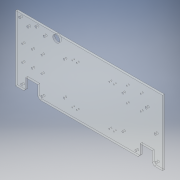
# Autodesk Inventor part: LexanPlatebkp
Saved by Autodesk Inventor 2018 (Build 220112000, 112)
## iProperties
Created: 2017-09-07
Part Number: LexanPlatebkp
Material: Polycarbonate, Clear
Document SubType Name: Modeling
Designer: Srinity
Density: 1.2 g/cm^3
Appearance: Polycarbonate - Clear
Author: Srinity
Autodesk Inventor part; units mm, degrees
ref_plane "YZ Plane" through (0, 0, 0) normal (1, 0, 0) x (0, 1, 0)
ref_plane "XZ Plane" through (0, 0, 0) normal (0, 1, 0) x (-1, 0, 0)
ref_plane "XY Plane" through (0, 0, 0) normal (0, 0, 1) x (1, 0, 0)
sketch "Sketch1" plane through (0, 0, 0) normal (0, 0, 1) x (1, 0, 0)
  line L0 (-228.6, 101.6) -> (228.6, 101.6)
  line L1 (228.6, 101.6) -> (228.6, -101.6)
  line L2 (228.6, -101.6) -> (-228.6, -101.6)
  line L3 (-228.6, -101.6) -> (-228.6, 101.6)
  point P0 (0, 0)
  dimension "d0" = 457.2
  dimension "d1" = 203.2
  dimension "d2" = 228.6
  dimension "d3" = 101.6
  constraints: 8 end point, 2 parallel, 1 horizontal, 1 perpendicular
  measures "d0" distance of L0.start L0.end
  measures "d1" distance of L2.end L0.start
  measures "d2" distance from line of point (0, 0) L3
  measures "d3" distance from line of point (0, 0) L0
extrude "Extrusion1" add sketch "Sketch1" along normal blind 6.35
sketch "Sketch2" plane through (0, 0, 6.35) normal (0, 0, 1) x (1, 0, 0)
  line L0 (-228.6, -101.6) -> (228.6, -101.6) projected
  line L1 (-196.85, -101.6) -> (-158.75, -101.6)
  line L2 (-158.75, -101.6) -> (-158.75, -63.5)
  line L3 (-158.75, -63.5) -> (-196.85, -63.5)
  line L4 (-196.85, -63.5) -> (-196.85, -101.6)
  line L5 (158.75, -101.6) -> (196.85, -101.6)
  line L6 (196.85, -101.6) -> (196.85, -63.5)
  line L7 (196.85, -63.5) -> (158.75, -63.5)
  line L8 (158.75, -63.5) -> (158.75, -101.6)
  line L9 (-228.6, 101.6) -> (-228.6, -101.6) projected
  line L10 (228.6, -101.6) -> (228.6, 101.6) projected
  point P0 (0, 0)
  dimension "d6" = 31.75
  dimension "d7" = 38.1
  dimension "d8" = 38.1
  dimension "d9" = 31.75
  constraints: 16 end point, 4 parallel, 2 equal length, 2 horizontal, 2 perpendicular, 2 point on line
  measures "d6" distance between parallel lines of L4 L9
  measures "d7" distance of L2.end L3.end
  measures "d8" distance of L1.end L2.end
  measures "d9" distance between parallel lines of L10 L6
extrude "Extrusion2" cut sketch "Sketch2" against normal through all
chamfer "Chamfer1" distance 6.35 angle 45 4 edges at (196.85, -101.6, 3.175) (158.75, -101.6, 3.175) (-196.85, -101.6, 3.175) (-158.75, -101.6, 3.175)
sketch "Sketch3" plane through (0, 0, 0) normal (0, 0, -1) x (-1, 0, 0)
  circle A0 centre (-209.55, -88.9) radius 3.175
  circle A1 centre (-146.05, -88.9) radius 3.175
  circle A2 centre (146.05, -88.9) radius 3.175
  circle A3 centre (209.55, -88.9) radius 3.175
  line L0 (-152.4, -101.6) -> (152.4, -101.6) projected
  line L1 (-228.6, 101.6) -> (-228.6, -101.6) projected
  line L2 (228.6, -101.6) -> (228.6, 101.6) projected
  point P0 (0, 0)
  dimension "d15" = 12.7
  dimension "d16" = 6.35
  dimension "d17" = 19.05
  dimension "d18" = 63.5
  dimension "d19" = 63.5
  dimension "d20" = 19.05
  constraints: 4 centre point, 3 equal radius, 3 horizontal alignment
  measures "d15" distance from line of A1.centre L0
  measures "d16" diameter of A1
  measures "d17" distance from line of A0.centre L1
  measures "d18" distance of A0.centre A1.centre
  measures "d19" distance of A3.centre A2.centre
  measures "d20" distance from line of L2 A3.centre
extrude "Extrusion3" cut sketch "Sketch3" against normal blind 25.4
sketch "Sketch4" plane through (0, 0, 0) normal (0, 0, -1) x (-1, 0, 0)
  circle A0 centre (139.7, 76.2) radius 3.302 projected
  circle A1 centre (165.1, 88.9) radius 3.302 projected
  circle A2 centre (190.5, 76.2) radius 3.302 projected
  circle A3 centre (215.9, 88.9) radius 3.302 projected
  circle A4 centre (147.0661, 22.2869) radius 2.513 projected
  circle A5 centre (177.1772, 22.2869) radius 2.513 projected
  circle A6 centre (207.2882, 22.2869) radius 2.513 projected
  circle A7 centre (207.2882, -28.5131) radius 2.513 projected
  circle A8 centre (177.1772, -28.5131) radius 2.5956 projected
  circle A9 centre (147.0661, -28.5131) radius 2.513 projected
  circle A10 centre (-77.3373, 55.245) radius 1.5428 projected
  circle A11 centre (52.0503, 55.245) radius 1.5428 projected
  circle A12 centre (52.0503, -71.4248) radius 1.5428 projected
  circle A13 centre (-77.3373, -71.4248) radius 1.5428 projected
  arc A14 (-104.9183, -56.1295) -> (-107.5853, -58.7965) centre (-104.9183, -58.7965) ccw projected
  arc A15 (-102.2513, -58.7965) -> (-104.9183, -56.1295) centre (-104.9183, -58.7965) ccw projected
  arc A16 (-104.9183, -61.4635) -> (-102.2513, -58.7965) centre (-104.9183, -58.7965) ccw projected
  arc A17 (-107.5853, -58.7965) -> (-104.9183, -61.4635) centre (-104.9183, -58.7965) ccw projected
  arc A18 (77.3521, -56.1295) -> (74.6851, -58.7965) centre (77.3521, -58.7965) ccw projected
  arc A19 (74.6851, -58.7965) -> (77.3521, -61.4635) centre (77.3521, -58.7965) ccw projected
  arc A20 (77.3521, -61.4635) -> (80.0191, -58.7965) centre (77.3521, -58.7965) ccw projected
  arc A21 (80.0191, -58.7965) -> (77.3521, -56.1295) centre (77.3521, -58.7965) ccw projected
  arc A22 (80.0191, 45.5975) -> (77.3521, 48.2645) centre (77.3521, 45.5975) ccw projected
  arc A23 (77.3521, 48.2645) -> (74.6851, 45.5975) centre (77.3521, 45.5975) ccw projected
  arc A24 (74.6851, 45.5975) -> (77.3521, 42.9305) centre (77.3521, 45.5975) ccw projected
  arc A25 (77.3521, 42.9305) -> (80.0191, 45.5975) centre (77.3521, 45.5975) ccw projected
  arc A26 (-104.9183, 42.9305) -> (-102.2513, 45.5975) centre (-104.9183, 45.5975) ccw projected
  arc A27 (-107.5853, 45.5975) -> (-104.9183, 42.9305) centre (-104.9183, 45.5975) ccw projected
  arc A28 (-104.9183, 48.2645) -> (-107.5853, 45.5975) centre (-104.9183, 45.5975) ccw projected
  arc A29 (-102.2513, 45.5975) -> (-104.9183, 48.2645) centre (-104.9183, 45.5975) ccw projected
  circle A30 centre (-160.782, 71.882) radius 1.905 projected
  circle A31 centre (-160.782, 24.13) radius 1.905 projected
  circle A32 centre (-117.729, 24.1324) radius 1.905 projected
  circle A33 centre (-117.729, 71.882) radius 1.905 projected
  circle A34 centre (146.05, -88.9) radius 3.175 projected
  circle A35 centre (-209.55, -88.9) radius 3.175 projected
  circle A36 centre (-146.05, -88.9) radius 3.175 projected
  circle A37 centre (209.55, -88.9) radius 3.175 projected
  line L0 (158.75, -95.25) -> (152.4, -101.6) projected
  line L1 (158.75, -95.25) -> (158.75, -63.5) projected
  line L2 (158.75, -63.5) -> (196.85, -63.5) projected
  line L3 (196.85, -63.5) -> (196.85, -95.25) projected
  line L4 (203.2, -101.6) -> (196.85, -95.25) projected
  line L5 (203.2, -101.6) -> (228.6, -101.6) projected
  line L6 (228.6, -101.6) -> (228.6, 101.6) projected
  line L7 (228.6, 101.6) -> (-228.6, 101.6) projected
  line L8 (-228.6, 101.6) -> (-228.6, -101.6) projected
  line L9 (-228.6, -101.6) -> (-203.2, -101.6) projected
  line L10 (-196.85, -95.25) -> (-203.2, -101.6) projected
  line L11 (-196.85, -95.25) -> (-196.85, -63.5) projected
  line L12 (-196.85, -63.5) -> (-158.75, -63.5) projected
  line L13 (-158.75, -63.5) -> (-158.75, -95.25) projected
  line L14 (-152.4, -101.6) -> (-158.75, -95.25) projected
  line L15 (-152.4, -101.6) -> (152.4, -101.6) projected
  circle A38 centre (-177.8, 42.5448) radius 3.429 projected
  circle A39 centre (-205.74, -14.6052) radius 3.429 projected
  point P0 (0, 0)
extrude "Extrusion4" cut sketch "Sketch4" against normal through all contours A0 | A1 | A2 | A3 | A4 | A5 | A6 | A7 | A8 | A9 | A10 | A11 | A12 | A13 | A15 A16 A17 A14 | A21 A20 A19 A18 | A25 A24 A23 A22 | A27 A28 A29 A26 | A30 | A31 | A32 | A33 | A38 | A39
sketch "Sketch5" plane through (0, 0, 6.35) normal (0, 0, 1) x (1, 0, 0)
  line L0 (-90.717, 90.4998) -> (-91.3, 90.4141) projected
  line L1 (-91.3, 90.4141) -> (-91.3, 87.3859) projected
  line L2 (-91.3, 87.3859) -> (-90.717, 87.3002) projected
  arc A0 (-112.483, 87.3002) -> (-90.717, 87.3002) centre (-101.6, 88.9) ccw projected
  line L3 (-112.483, 87.3002) -> (-111.9, 87.3859) projected
  line L4 (-111.9, 87.3859) -> (-111.9, 90.4141) projected
  line L5 (-111.9, 90.4141) -> (-112.483, 90.4998) projected
  arc A1 (-103.0998, 99.7973) -> (-112.483, 90.4998) centre (-101.6, 88.9) ccw projected
  line L6 (-103.1, 101.3) -> (-103.0998, 99.7973) projected
  line L7 (-103.1, 101.3) -> (-100.1, 101.3) projected
  line L8 (-100.1002, 99.7973) -> (-100.1, 101.3) projected
  arc A2 (-90.717, 90.4998) -> (-100.1002, 99.7973) centre (-101.6, 88.9) ccw projected
  circle A3 centre (-101.6, 88.9) radius 17.9999 projected
  circle A4 centre (-101.6, 88.9) radius 11
  point P0 (0, 0)
  constraints: 1 centre point, 1 coincident, 1 concentric
extrude "Extrusion5" cut sketch "Sketch5" against normal through all contours A4 L2 L1 L0 | L0 L1 L2 A0 L3 L4 L5 A1 A4 A2 | L5 L4 L3 A4
sketch "Sketch6" plane through (0, 0, 6.35) normal (0, 0, 1) x (1, 0, 0)
  circle A0 centre (-38.1565, 55.4101) radius 1.8832
  circle A1 centre (63.4435, 55.4101) radius 1.8832
  circle A2 centre (63.4435, -71.5899) radius 1.8832
  circle A3 centre (-38.1565, -71.5899) radius 1.8832
  point P0 (0, 0)
  constraints: 4 centre point, 8 other
extrude "Extrusion6" cut sketch "Sketch6" against normal blind 25.4
equation "\"d2\" = 0.5 * d0"
equation "\"d3\" = 0.5 * d1"
equation "\"d9\" = d6"
equation "\"d19\" = d18"
equation "\"d20\" = d17"
body "Solid1"
